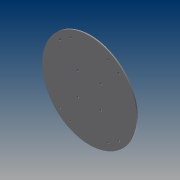
# Autodesk Inventor part: BaseBottom
Saved by Autodesk Inventor 2011 SP1 (Build 150282100, 282)
## iProperties
Created: 2011-07-18
Part Number: BaseBottom
Document SubType Name: Modeling
Designer: Nathan
Density: 1 g/cm^3
Mass: 24.3438 g
Surface Area: 315.367 cm^2
Volume: 24.3438 cm^3
Author: Nathan
Autodesk Inventor part; units mm, degrees
ref_plane "YZ Plane" through (0, 0, 0) normal (1, 0, 0) x (0, 1, 0)
ref_plane "XZ Plane" through (0, 0, 0) normal (0, 1, 0) x (-1, 0, 0)
ref_plane "XY Plane" through (0, 0, 0) normal (0, 0, 1) x (1, 0, 0)
sketch "Sketch1" plane through (0, 0, 0) normal (0, 0, 1) x (1, 0, 0)
  line L0 (0, 10.0078) -> (0, -10.7712)
  line L1 (-20.5368, 0) -> (25.7294, 0)
  line L2 (0, 0) -> (-9.8402, -9.8402)
  line L3 (0, 0) -> (13.9161, 0) construction
  line L4 (0, 0) -> (-23.2805, 23.2805)
  circle A0 centre (0, 0) radius 66.675
  point P0 (-16.1645, 16.1645)
  point P1 (-41.3092, 41.3092)
  point P2 (-41.3092, -41.3092)
  point P3 (-16.1645, -16.1645)
  point P4 (16.1645, 16.1645)
  point P5 (41.3092, 41.3092)
  point P6 (41.3092, -41.3092)
  point P7 (16.1645, -16.1645)
  point P8 (26.5906, 50.8)
  point P9 (-26.5906, 50.8)
  point P10 (23.2805, 23.2805)
  point P11 (16.1645, 16.1645)
  point P12 (26.5906, -50.8)
  point P13 (-26.5906, -50.8)
  dimension "d1" = 45
  dimension "d56" = 22.86
  dimension "d58" = 35.56
  dimension "d67" = 53.1812
  dimension "d68" = 101.6
  dimension "d85" = 133.35
  constraints: 11 symmetric about line, 10 end point, 2 horizontal, 2 perpendicular, 2 point on line, 2 vertical, 1 centre point, 1 coincident, 1 equal length
  measures "d1" angle of L3 L2
  measures "d56" distance of L2.start point (-16.164, 16.164)
  measures "d58" distance of point (-41.309, 41.309) point (-16.164, 16.164)
  measures "d67" distance of point (-26.591, -50.8) point (26.591, -50.8)
  measures "d68" distance of point (26.591, -50.8) point (26.591, 50.8)
  measures "d85" diameter of A0
extrude "Extrusion1" add sketch "Sketch1" along normal blind 1.5875
hole "Hole1" at (-16.1645, 16.1645, 0) at (-41.3092, 41.3092, 0) at (-41.3092, -41.3092, 0) at (-16.1645, -16.1645, 0) at (41.3092, 41.3092, 0) at (16.1645, 16.1645, 0) at (16.1645, -16.1645, 0) at (41.3092, -41.3092, 0) direction (0, 0, 1) diameter 3.302 end through all thread size "8-32 UNC" class "2B" standard "ANSI Unified Screw Threads"
sketch "Sketch2" plane through (0, 0, 0) normal (0, 0, -1) x (-1, 0, 0)
  line L0 (0, -11.8713) -> (0, 16.3095)
  line L1 (-16.3095, 0) -> (16.3095, 0)
  point P0 (23.2805, -60.3987)
  point P1 (0, 0)
  point P2 (26.5906, 50.8)
  point P3 (-26.5906, 50.8)
  point P4 (26.5906, -50.8)
  point P5 (-26.5906, -50.8)
  dimension "d69" = 53.1812
  dimension "d70" = 101.6
  constraints: 4 end point, 3 symmetric about line, 2 vertical, 1 horizontal, 1 perpendicular
  measures "d69" distance of point (-26.591, -50.8) point (26.591, -50.8)
  measures "d70" distance of point (26.591, -50.8) point (26.591, 50.8)
hole "Hole3" at (-26.5906, -50.8, 0) at (26.5906, -50.8, 0) at (26.5906, 50.8, 0) at (-26.5906, 50.8, 0) direction (0, 0, 1) diameter 2.6416 end through all thread size "6-32 UNC" class "2B" standard "ANSI Unified Screw Threads"
body "Solid1"
